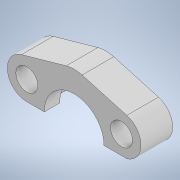
# Autodesk Inventor part: 50073 Полуфланец
Saved by Autodesk Inventor 2021 (Build 250183000, 183)
## iProperties
Created: 2021-03-02
Part Number: 50073 Полуфланец
Material: Типовые
Document SubType Name: Modeling
Designer: mrily
Density: 1 g/cm^3
Appearance: По умолчанию
Author: mrily
Autodesk Inventor part; units mm, degrees
ref_plane "YZ Plane" through (0, 0, 0) normal (1, 0, 0) x (0, 1, 0)
ref_plane "XZ Plane" through (0, 0, 0) normal (0, 1, 0) x (-1, 0, 0)
ref_plane "XY Plane" through (0, 0, 0) normal (0, 0, 1) x (1, 0, 0)
sketch "Эскиз1" plane through (0, 0, 0) normal (0, 0, 1) x (1, 0, 0)
  line L0 (0, 18.7367) -> (0, -24.5413)
  arc A0 (21.6223, -7.6994) -> (21.6223, 7.6994) centre (19.45, 0) ccw
  line L1 (19.45, 0) -> (21.6223, -7.6994) construction
  line L2 (19.45, 0) -> (17.2777, 7.6994) construction
  arc A1 (-21.6223, 7.6994) -> (-19.45, -8) centre (-19.45, 0) ccw
  line L3 (-19.45, 0) -> (-19.45, 7.9959) construction
  line L4 (-19.45, 0) -> (-11.4541, 0) construction
  line L5 (-19.45, 0) -> (-19.45, -8) construction
  arc A2 (12.25, -7.6994) -> (-12.2463, -8) centre (0, -7.6994) ccw
  line L6 (-21.6223, 7.6994) -> (-3.2585, 12.8806)
  line L7 (3.2585, 12.8806) -> (21.6223, 7.6994)
  line L8 (21.6223, -7.6994) -> (12.25, -7.6994)
  line L9 (-19.45, -8) -> (-12.2463, -8)
  circle A3 centre (-19.45, 0) radius 4.5
  circle A4 centre (19.45, 0) radius 4.5
  arc A5 (3.2585, 12.8806) -> (-3.2585, 12.8806) centre (0, 1.3315) ccw
  point P0 (0, 0)
  point P1 (-27.45, 0)
  point P2 (27.45, 0)
  point P3 (0, 13.8)
  dimension "d0" = 8
  dimension "d1" = 180
  dimension "d3" = 8
  dimension "d4" = 90
  dimension "d5" = 180
  dimension "d6" = 24.5
  dimension "d7" = 54.9
  dimension "d9" = 21.8
  dimension "d10" = 9
  dimension "d11" = 9
  dimension "d12" = 12
  constraints: 20 end point, 10 point on circle, 6 centre point, 5 horizontal alignment, 5 point on line, 4 tangent, 3 horizontal, 2 coincident, 2 equal length, 1 vertical
  measures "d0" radius of A0
  measures "d1" angle of L2 L1
  measures "d3" radius of A1
  measures "d4" angle of L4 L3
  measures "d5" angle of L3 L5
  measures "d6" diameter of A2
  measures "d7" distance of point (-27.45, 0) point (27.45, 0)
  measures "d9" vertical distance of L5.end point (0, 13.8)
  measures "d10" diameter of A3
  measures "d11" diameter of A4
  measures "d12" radius of A5
extrude "Выдавливание1" add sketch "Эскиз1" against normal blind 13
sketch "Эскиз2" plane through (0, 0, -13) normal (0, 0, -1) x (-1, 0, 0)
  circle A0 centre (0, -8) radius 15.475
  point P0 (0, 0)
  point P1 (12.2463, -8)
  dimension "d15" = 30.95
  constraints: 1 centre point, 1 horizontal alignment, 1 vertical alignment
  measures "d15" diameter of A0
extrude "Выдавливание2" cut sketch "Эскиз2" against normal blind 6.2
fillet "Сопряжение1" radius 0.5 1 edges at (-0.1503, 7.4743, -6.8)
chamfer "Фаска1" distance 0.5 angle 45 1 edges at (-0.1503, 7.4743, -13) measured on face at (-11.2492, 8.421, -13)
chamfer "Фаска2" distance 0.5 angle 45 1 edges at (-0.1503, 4.5497, -6.8) measured on face at (13.8976, -6.5154, -6.8)
